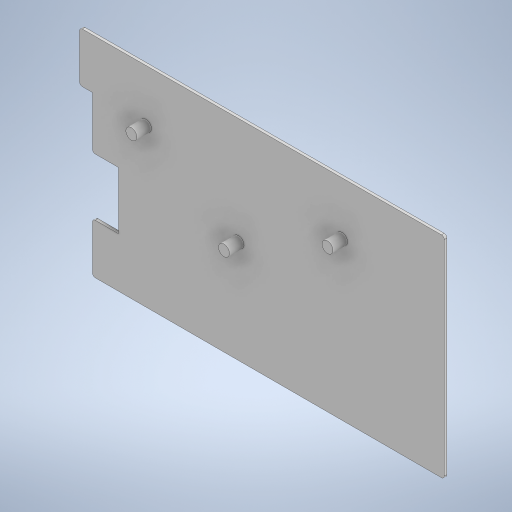
# Autodesk Inventor part: BottomInner_right
Saved by Autodesk Inventor 2023 (Build 270158000, 158)
## iProperties
Created: 2022-11-25
Part Number: BottomInner_right
Material: Generic
Document SubType Name: Modeling
Designer: reide
Density: 1 g/cm^3
Appearance: Default
Author: reide
Autodesk Inventor part; units mm, degrees
ref_plane "YZ Plane" through (0, 0, 0) normal (1, 0, 0) x (0, 1, 0)
ref_plane "XZ Plane" through (0, 0, 0) normal (0, 1, 0) x (-1, 0, 0)
ref_plane "XY Plane" through (0, 0, 0) normal (0, 0, 1) x (1, 0, 0)
sketch "Sketch1" plane through (0, 0, 0) normal (0, 0, 1) x (1, 0, 0)
  line L0 (67.175, 38.35) -> (67.175, 15.986)
  arc A0 (67.175, 38.35) -> (66.175, 39.35) centre (66.175, 38.35) ccw
  line L1 (-33.175, 39.35) -> (66.175, 39.35)
  arc A1 (-34.175, 40.35) -> (-33.175, 39.35) centre (-33.175, 40.35) ccw
  line L2 (-34.175, 40.35) -> (-34.175, 43.6)
  line L3 (-34.175, 43.6) -> (-34.5505, 43.6)
  spline S0 degree 3 poles (-35.175, 43.605) (-35.038, 43.605) (-34.8736, 43.6028) (-34.6784, 43.6006) (-34.6086, 43.6) (-34.5505, 43.6) knots 0 0 0 0 0.702117 0.702117 1 1 1 1
  line L4 (-51.175, 43.605) -> (-35.175, 43.605)
  spline S1 degree 3 poles (-51.7995, 43.6) (-51.7414, 43.6) (-51.6716, 43.6006) (-51.4764, 43.6028) (-51.312, 43.605) (-51.175, 43.605) knots 0 0 0 0 0.297883 0.297883 1 1 1 1
  line L5 (-51.7995, 43.6) -> (-52.175, 43.6)
  line L6 (-52.175, 43.6) -> (-52.175, 40.35)
  arc A2 (-53.175, 39.35) -> (-52.175, 40.35) centre (-53.175, 40.35) ccw
  line L7 (-67.175, 39.35) -> (-53.175, 39.35)
  line L8 (-67.175, 20.05) -> (-67.175, 39.35)
  line L9 (-62.412, 20.05) -> (-67.175, 20.05)
  line L10 (-62.412, 1) -> (-62.412, 20.05)
  line L11 (-52.887, 1) -> (-62.412, 1)
  line L12 (-52.887, -20.05) -> (-52.887, 1)
  line L13 (-62.4125, -20.05) -> (-52.887, -20.05)
  line L14 (-62.4125, -39.35) -> (-62.4125, -20.05)
  line L15 (66.175, -39.35) -> (-62.4125, -39.35)
  arc A3 (66.175, -39.35) -> (67.175, -38.35) centre (66.175, -38.35) ccw
  line L16 (67.175, 0.986) -> (67.175, -38.35)
  arc A4 (68.175, 1.986) -> (67.175, 0.986) centre (68.175, 0.986) ccw
  line L17 (68.175, 1.986) -> (71.425, 1.986)
  line L18 (71.425, 1.986) -> (71.425, 2.3615)
  spline S2 degree 3 poles (71.43, 2.986) (71.43, 2.849) (71.4278, 2.6846) (71.4256, 2.4894) (71.425, 2.4196) (71.425, 2.3615) knots 0 0 0 0 0.702117 0.702117 1 1 1 1
  line L19 (71.43, 13.986) -> (71.43, 2.986)
  spline S3 degree 3 poles (71.425, 14.6105) (71.425, 14.5524) (71.4256, 14.4826) (71.4278, 14.2874) (71.43, 14.123) (71.43, 13.986) knots 0 0 0 0 0.297883 0.297883 1 1 1 1
  line L20 (71.425, 14.6105) -> (71.425, 14.986)
  line L21 (71.425, 14.986) -> (68.175, 14.986)
  arc A5 (67.175, 15.986) -> (68.175, 14.986) centre (68.175, 15.986) ccw
  line L22 (-67.175, 39.35) -> (-67.175, 38.35)
  line L23 (-67.175, 39.35) -> (67.175, 39.35)
  line L24 (67.175, 39.35) -> (67.175, -39.35)
  line L25 (67.175, -39.35) -> (-67.175, -39.35)
  line L26 (-67.175, -39.35) -> (-67.175, 39.35)
  line L27 (67.175, -39.35) -> (67.175, -38.35)
  line L28 (67.175, -38.35) -> (-62.4125, -38.35)
  line L29 (67.175, 39.35) -> (67.175, 38.85)
  line L30 (67.175, 38.85) -> (-67.175, 38.35)
  line L31 (67.175, 39.35) -> (66.675, 39.35)
  line L32 (66.675, 39.35) -> (67.175, 39.35)
  line L33 (67.175, 39.35) -> (67.175, -39.35)
  line L34 (67.175, -39.35) -> (66.675, -39.35)
  line L35 (66.675, -39.35) -> (66.675, 39.35)
  point P0 (0, 0)
  point P1 (67.175, -38.35)
  point P2 (67.0413, 38.8495)
  point P3 (66.675, -38.35)
  point P4 (66.675, 38.8481)
  dimension "d0" = 1
  dimension "d1" = 1
  dimension "d2" = 0.5
  dimension "d16" = 0.5
  constraints: 28 end point, 5 point on line, 4 parallel, 3 perpendicular, 2 horizontal
  measures "d0" distance of L7.start L22.end
  measures "d1" distance of L24.end L27.end
  measures "d2" distance of L23.end L29.end
  measures "d16" distance of L23.end L31.end
extrude "Extrusion1" add sketch "Sketch1" along normal blind 1 contours L35 L28 L14 L13 L12 L11 L10 L9 L8 L30
fillet "Fillet1" radius 1 7 edges at (-67.175, 38.35, 0.5) (-67.175, 20.05, 0.5) (-62.412, 1, 0.5) (-62.4125, -20.05, 0.5) (-62.4125, -38.35, 0.5) (66.675, 38.8481, 0.5) (66.675, -38.35, 0.5)
sketch "Sketch2" plane through (0, 0, 1) normal (0, 0, 1) x (1, 0, 0)
  line L0 (65.6713, 38.8444) -> (-66.1787, 38.3537) projected
  arc A0 (-66.1787, 38.3537) -> (-67.175, 37.3537) centre (-66.175, 37.3537) ccw projected
  line L1 (-67.175, 37.3537) -> (-67.175, 21.05) projected
  arc A1 (-67.175, 21.05) -> (-66.175, 20.05) centre (-66.175, 21.05) ccw projected
  line L2 (-66.175, 20.05) -> (-62.412, 20.05) projected
  line L3 (-62.412, 20.05) -> (-62.412, 2) projected
  arc A2 (-62.412, 2) -> (-61.412, 1) centre (-61.412, 2) ccw projected
  line L4 (-61.412, 1) -> (-52.887, 1) projected
  line L5 (-52.887, 1) -> (-52.887, -20.05) projected
  line L6 (-52.887, -20.05) -> (-61.4125, -20.05) projected
  arc A3 (-61.4125, -20.05) -> (-62.4125, -21.05) centre (-61.4125, -21.05) ccw projected
  line L7 (-62.4125, -21.05) -> (-62.4125, -37.35) projected
  arc A4 (-62.4125, -37.35) -> (-61.4125, -38.35) centre (-61.4125, -37.35) ccw projected
  line L8 (-61.4125, -38.35) -> (65.675, -38.35) projected
  line L9 (67.175, 38.85) -> (67.175, 19.35)
  line L10 (67.175, 19.35) -> (29.175, 19.35)
  circle A5 centre (29.175, 19.35) radius 2
  line L11 (29.175, 19.35) -> (-42.825, 19.35)
  circle A6 centre (-42.825, 19.35) radius 2
  line L12 (29.175, 19.35) -> (-8.825, 19.35)
  line L13 (-8.825, 19.35) -> (-8.825, -0.65)
  circle A7 centre (-8.825, -0.65) radius 2
  line L14 (66.675, -37.35) -> (66.675, 37.8444) projected
  arc A8 (65.675, -38.35) -> (66.675, -37.35) centre (65.675, -37.35) ccw projected
  arc A9 (66.675, 37.8444) -> (65.6713, 38.8444) centre (65.675, 37.8444) ccw projected
  point P0 (0, 0)
  dimension "d6" = 19.5
  dimension "d7" = 38
  dimension "d8" = 4
  dimension "d9" = 72
  dimension "d10" = 4
  dimension "d11" = 38
  dimension "d12" = 20
  dimension "d13" = 4
  constraints: 10 end point, 3 centre point, 3 coincident, 1 horizontal, 1 perpendicular, 1 point on line
  measures "d6" distance of L9.start L9.end
  measures "d7" distance of L9.end L10.end
  measures "d8" diameter of A5
  measures "d9" distance of L11.start L11.end
  measures "d10" diameter of A6
  measures "d11" distance of L11.start L12.end
  measures "d12" distance of L12.end L13.end
  measures "d13" diameter of A7
extrude "Extrusion2" add sketch "Sketch2" along normal blind 5.35 contours A5 L11 L10 | L10 L11 A5 | A6 | A7
body "Solid1"
